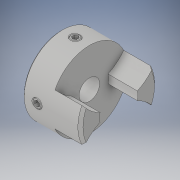
# Autodesk Inventor part: MJT-30-BL-8-12 Hub 1
Saved by Autodesk Inventor 2019 (Build 230136000, 136)
## iProperties
Created: 2023-09-29
Part Number: MJT-30-BL-8-12 Hub 1
Material: Generic
Catalog Web Link: www.cadenas.de
Description: MJT Hub 1-
Vendor: NBK
Document SubType Name: Modeling
Designer: psAdmin
Manufacturer: NBK
Mass: 8.48055 g
Surface Area: 34.4763 cm^2
Volume: 8.48055 cm^3
Density: 1 g/cm^3
Appearance: PSOLRGB-175-175-175
Category: PARTsolutions
Company: NBK
Title: MJT-30-BL-8-12 Hub 1
Author: Cadenas PARTsolutions
PSOL_IDENT_0: {$CADENAS_DATA/23d-libs/nbk/motion_control_parts/couplicon_mini/jaw_type/mjt/mjt_1.prj},187 {VTYP=3D
PSOL_IDENT_1: },{NB=MJT-30-BL-8-12 Hub 1},{LINA=MJT-30-BL-8-12 Hub 1},{NN=MJT Hub 1},{DATE=25.09.2023 00:41:45},{G
PSOL_IDENT_2: EOMDATE=30.03.2016 02:13:22},{VERSION=},{LINEID=30},{WBVAR=D1D2},{WBNUMERIC=}  {NB=MJT-30-BL-8-12 Hu
PSOL_IDENT_3: b 1},{LINA=MJT-30-BL-8-12 Hub 1},{KT=DUMMY},{CN=MJT-30-BL},{D1D2=8-12},{D1D2X1='6-6','6-6.35','6-7','
PSOL_IDENT_4: 6-8','6-9.525','6-10','6-11','6-12','6-14','6-15','6-16','6.35-6.35','6.35-7','6.35-8','6.35-9.525','
PSOL_IDENT_5: 6.35-10','6.35-11','6.35-12','6.35-14','6.35-15','6.35-16','7-7','7-8','7-9.525','7-10','7-11','7-12'
PSOL_IDENT_6: ,'7-14','7-15','7-16','8-8','8-9.525','8-10','8-11','8-12','8-14','8-15','8-16','9.525-9.525','9.525
PSOL_IDENT_7: -10','9.525-11','9.525-12','9.525-14','9.525-15','9.525-16','10-10','10-11','10-12','10-14','10-15','
PSOL_IDENT_8: 10-16','11-11','11-12','11-14','11-15','11-16','12-12','12-14','12-15','12-16','14-14','14-15','14-1
PSOL_IDENT_9: 6','15-15','15-16','16-16'},{TEST='6x6','6x6.35','6x7','6x8','6x9.525','6x10','6x11','6x12','6x14','
PSOL_IDENT_10: 6x15','6x16','6.35x6.35','6.35x7','6.35x8','6.35x9.525','6.35x10','6.35x11','6.35x12','6.35x14','6.3
PSOL_IDENT_11: 5x15','6.35x16','7x7','7x8','7x9.525','7x10','7x11','7x12','7x14','7x15','7x16','8x8','8x9.525','8x1
PSOL_IDENT_12: 0','8x11','8x12','8x14','8x15','8x16','9.525x9.525','9.525x10','9.525x11','9.525x12','9.525x14','9.5
PSOL_IDENT_13: 25x15','9.525x16','10x10','10x11','10x12','10x14','10x15','10x16','11x11','11x12','11x14','11x15','1
PSOL_IDENT_14: 1x16','12x12','12x14','12x15','12x16','14x14','14x15','14x16','15x15','15x16','16x16'},{VERS=1},{YV=
PSOL_IDENT_15: 0.5},{YU=1.0},{A=30},{L=11},{W=35},{B=10},{C=1.5},{F=5.5},{M=M4},{KDMM=3.242},{NDM=4.00},{KDMV=3.141
PSOL_IDENT_16: },{DV=7.00},{D1=8},{D2=12},{DP=13.22},{DP1=0.00},{RV=1.500},{S=2.0}
NB: MJT-30-BL-8-12 Hub 1
NN: MJT Hub 1
NBSYN: $CN.-$D1D2. Hub 1
LINA: MJT-30-BL-8-12 Hub 1
CATALOG: NBK (Nabeya Bi-tech Kaisha
CN: MJT-30-BL
D1D2: 8-12
D1D2X1: '6-6','6-6.35','6-7','6-8','6-9.525','6-10','6-11','6-12','6-14','6-15','6-16','6.35-6.35','6.35-7','6.35-8','6.35-9.525','6.35-10','6.35-11','6.35-12','6.35-14','6.35-15','6.35-16','7-7','7-8','7-9.525','7-10','7-11','7-12','7-14','7-15','7-16','8-8','8-9.525','8-10','8-11','8-12','8-14','8-15','8-16','9.525-9.525','9.525-10','9.525-11','9.525-12','9.525-14','9.525-15','9.525-16','10-10','10-11','10-12','10-14','10-15','10-16','11-11','11-12','11-14','11-15','11-16','12-12','12-14','12-15','12-16','14-14','14-15','14-16','15-15','15-16','16-16'
VERS: 1
YV: 0.5
YU: 1
A: 30
L: 11
W: 35
B: 10
C: 1.5
F: 5.5
M: M4
KDMM: 3.242
NDM: 4
KDMV: 3.141
DV: 7
DP: 13.22
DP1: 0
RV: 1.5
S: 2
SUPPLIER: NBK
ARTICLENO: MJT-30-BL-8-12 Hub 1
BOMINFO: MJT-30-BL-8-12 Hub 1
CREATOR: CADENAS GmbH
Autodesk Inventor part; units mm, degrees
sketch "Sketch_1" plane through (0, 0, 0) normal (0, 0, 1) x (1, 0, 0)
  line L0 (22.5, 0) -> (0, 0)
  line L1 (0, 14.5) -> (0, 4)
  line L2 (0, 4) -> (22.5, 4)
  line L3 (22.5, 4) -> (22.5, 14)
  line L4 (22.5, 14) -> (21.5, 15)
  line L5 (21.5, 15) -> (0.5, 15)
  line L6 (0.5, 15) -> (0, 14.5)
  constraints: 14 end point
revolve "Revolution1" add sketch "Sketch_1" angle 360 about axis through (22.5, 0, 0) along (1, 0, 0)
sketch "Sketch_2" plane through (11, 0, 0) normal (1, 0, 0) x (0, 0, -1)
  arc A0 (-13.4651, -6.61) -> (13.4651, -6.61) centre (0, 0) ccw
  arc A1 (13.4651, -6.61) -> (7.3157, -1.6525) centre (0, -17.0197) ccw
  arc A2 (7.3157, -1.6525) -> (7.3157, 1.6525) centre (0, 0) ccw
  arc A3 (7.3157, 1.6525) -> (13.4651, 6.61) centre (0, 17.0197) ccw
  arc A4 (13.4651, 6.61) -> (-13.4651, 6.61) centre (0, 0) ccw
  arc A5 (-13.4651, 6.61) -> (-7.3157, 1.6525) centre (0, 17.0197) ccw
  arc A6 (-7.3157, 1.6525) -> (-7.3157, -1.6525) centre (0, 0) ccw
  arc A7 (-7.3157, -1.6525) -> (-13.4651, -6.61) centre (0, -17.0197) ccw
  constraints: 16 point on circle, 8 centre point
extrude "Extrusion1" cut sketch "Sketch_2" along normal blind 11.5
sketch "Sketch_7" plane through (0, 0, 0) normal (0, 0, 1) x (1, 0, 0)
  line L0 (5.5, 0) -> (5.5, 15)
  line L1 (5.5, 15) -> (7.5, 15)
  line L2 (7.5, 15) -> (7.121, 14.621)
  line L3 (7.121, 14.621) -> (7.121, 0.379)
  line L4 (7.121, 0.379) -> (7.5, 0)
  line L5 (7.5, 0) -> (5.5, 0)
  line L6 (5.5, 0) -> (5.5, 15)
  constraints: 14 end point
revolve "Revolution2" cut sketch "Sketch_7" angle 360 about axis through (5.5, 0, 0) along (0, -1, 0)
sketch "Sketch_8" plane through (0, 0, 0) normal (0, 1, 0) x (-1, 0, 0)
  line L0 (-5.5, 15) -> (-5.5, 0)
  line L1 (-5.5, 0) -> (-7.5, 0)
  line L2 (-7.5, 0) -> (-7.121, 0.379)
  line L3 (-7.121, 0.379) -> (-7.121, 14.621)
  line L4 (-7.121, 14.621) -> (-7.5, 15)
  line L5 (-7.5, 15) -> (-5.5, 15)
  line L6 (-5.5, 15) -> (-5.5, 0)
  constraints: 14 end point
revolve "Revolution3" cut sketch "Sketch_8" angle 360 about axis through (5.5, 0, 15) along (0, 0, 1)
sketch "Sketch_12" plane through (0, 0, 0) normal (0, 0, 1) x (1, 0, 0)
  line L0 (5.5, 8) -> (5.5, 15)
  line L1 (5.5, 15) -> (7.0705, 15)
  line L2 (7.0705, 15) -> (7.5, 14.5705)
  line L3 (7.5, 14.5705) -> (7.5, 8.4295)
  line L4 (7.5, 8.4295) -> (7.0705, 8)
  line L5 (7.0705, 8) -> (5.5, 8)
  line L6 (5.5, 8) -> (5.5, 15)
  constraints: 14 end point
revolve "Revolution4" add sketch "Sketch_12" angle 360 about axis through (5.5, 8, 0) along (0, -1, 0)
sketch "Sketch_13" plane through (0, 0, 0) normal (0, 1, 0) x (-1, 0, 0)
  line L0 (-5.5, 15) -> (-5.5, 8)
  line L1 (-5.5, 8) -> (-7.0705, 8)
  line L2 (-7.0705, 8) -> (-7.5, 8.4295)
  line L3 (-7.5, 8.4295) -> (-7.5, 14.5705)
  line L4 (-7.5, 14.5705) -> (-7.0705, 15)
  line L5 (-7.0705, 15) -> (-5.5, 15)
  line L6 (-5.5, 15) -> (-5.5, 8)
  constraints: 14 end point
revolve "Revolution5" add sketch "Sketch_13" angle 360 about axis through (5.5, 0, 15) along (0, 0, 1)
sketch "Sketch_14" plane through (0, 13.5, 0) normal (0, 1, 0) x (1, 0, 0)
  line L0 (4.5, -0.5774) -> (5.5, -1.1547)
  line L1 (5.5, -1.1547) -> (6.5, -0.5774)
  line L2 (6.5, -0.5774) -> (6.5, 0.5774)
  line L3 (6.5, 0.5774) -> (5.5, 1.1547)
  line L4 (5.5, 1.1547) -> (4.5, 0.5774)
  line L5 (4.5, 0.5774) -> (4.5, -0.5774)
  constraints: 12 end point
extrude "Extrusion2" cut sketch "Sketch_14" along normal blind 1.5
sketch "Sketch_15" plane through (0, 0, 13.5) normal (0, 0, 1) x (1, 0, 0)
  line L0 (4.5, -0.5774) -> (5.5, -1.1547)
  line L1 (5.5, -1.1547) -> (6.5, -0.5774)
  line L2 (6.5, -0.5774) -> (6.5, 0.5774)
  line L3 (6.5, 0.5774) -> (5.5, 1.1547)
  line L4 (5.5, 1.1547) -> (4.5, 0.5774)
  line L5 (4.5, 0.5774) -> (4.5, -0.5774)
  constraints: 12 end point
extrude "Extrusion3" cut sketch "Sketch_15" along normal blind 1.5
ref_plane "part1a_XY" through (0, 0, 0) normal (1, 0, 0) x (0, 0, -1)
ref_plane "part1a_YZ" through (0, 0, 0) normal (0, 0, -1) x (0, 1, 0)
ref_plane "part1a_ZX" through (0, 0, 0) normal (0, 1, 0) x (1, 0, 0)
ref_plane "part1b_XY" through (12.5, 0, 0) normal (1, 0, 0) x (0, 0, -1)
ref_plane "part1b_YZ" through (12.5, 0, 0) normal (0, 0, -1) x (0, 1, 0)
ref_plane "part1b_ZX" through (12.5, 0, 0) normal (0, 1, 0) x (1, 0, 0)
ref_plane "part1c_XY" through (22.5, 0, 0) normal (1, 0, 0) x (0, 0, -1)
ref_plane "part1c_YZ" through (22.5, 0, 0) normal (0, 0, -1) x (0, 1, 0)
ref_plane "part1c_ZX" through (22.5, 0, 0) normal (0, 1, 0) x (1, 0, 0)
body "Solid1"
